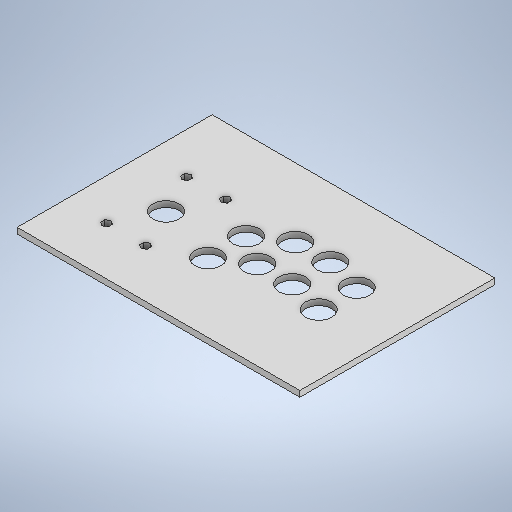
# Autodesk Inventor part: sega_straight_b1_v2
Saved by Autodesk Inventor 2025 (Build 290162010, 162A)
## iProperties
Created: 2022-12-25
Part Number: sega_straight_b1_v2
Material: Generic
Document SubType Name: Modeling
Designer: Bunny
Density: 1 g/cm^3
Appearance: Default
Author: Bunny
Autodesk Inventor part; units mm, degrees
ref_plane "YZ Plane" through (0, 0, 0) normal (1, 0, 0) x (0, 1, 0)
ref_plane "XZ Plane" through (0, 0, 0) normal (0, 1, 0) x (-1, 0, 0)
ref_plane "XY Plane" through (0, 0, 0) normal (0, 0, 1) x (1, 0, 0)
sketch "Sketch1" plane through (0, 0, 0) normal (0, 1, 0) x (-1, 0, 0)
  line L0 (145, -100) -> (-145, -100)
  line L1 (-145, -100) -> (-145, 100)
  line L2 (-145, 100) -> (145, 100)
  line L3 (145, 100) -> (145, -100)
  line L4 (210, 0) -> (-210, 0) projected
  line L5 (0, -140) -> (0, 140) projected
  point P0 (0, 0)
  dimension "d30" = 290
  dimension "d31" = 200
  constraints: 8 end point, 2 parallel, 1 horizontal, 1 perpendicular, 2 other
  measures "d30" distance of L0.start L0.end
  measures "d31" distance of L0.end L1.end
extrude "Extrusion1" add sketch "Sketch1" along normal blind 6
sketch "Sketch2" plane through (0, 6, 0) normal (0, 1, 0) x (1, 0, 0)
  circle A0 centre (-19.75, -29.5) radius 13.5
  circle A1 centre (-82.75, -9.5) radius 13.5
  circle A2 centre (-19.75, 9.5) radius 13.5
  circle A3 centre (46.75, 29.5) radius 13.5
  circle A4 centre (82.75, 20.5) radius 13.5
  circle A5 centre (10.75, 29.5) radius 13.5
  circle A6 centre (10.75, -9.5) radius 13.5
  circle A7 centre (46.75, -9.5) radius 13.5
  circle A8 centre (82.75, -18.5) radius 13.5
  line L0 (-96.25, 43) -> (96.25, 43)
  line L1 (96.25, 43) -> (96.25, -43)
  line L2 (96.25, -43) -> (-96.25, -43)
  line L3 (-96.25, -43) -> (-96.25, 43)
  line L4 (145, 100) -> (-145, 100) projected
  line L5 (145, -100) -> (145, 100) projected
  line L6 (0, 140) -> (0, -140) projected
  line L7 (-210, 0) -> (210, 0) projected
  line L8 (-102.75, 31.5) -> (-62.75, 31.5)
  line L9 (-62.75, 31.5) -> (-62.75, -50.5)
  line L10 (-62.75, -50.5) -> (-102.75, -50.5)
  line L11 (-102.75, -50.5) -> (-102.75, 31.5)
  line L12 (-106.75, 33.8094) -> (-102.75, 36.1188)
  line L13 (-102.75, 36.1188) -> (-98.75, 33.8094)
  line L14 (-98.75, 33.8094) -> (-98.75, 29.1906)
  line L15 (-98.75, 29.1906) -> (-102.75, 26.8812)
  line L16 (-102.75, 26.8812) -> (-106.75, 29.1906)
  line L17 (-106.75, 29.1906) -> (-106.75, 33.8094)
  line L18 (-62.75, 36.1188) -> (-58.75, 33.8094)
  line L19 (-58.75, 33.8094) -> (-58.75, 29.1906)
  line L20 (-58.75, 29.1906) -> (-62.75, 26.8812)
  line L21 (-62.75, 26.8812) -> (-66.75, 29.1906)
  line L22 (-66.75, 29.1906) -> (-66.75, 33.8094)
  line L23 (-66.75, 33.8094) -> (-62.75, 36.1188)
  line L24 (-102.75, -45.8812) -> (-98.75, -48.1906)
  line L25 (-98.75, -48.1906) -> (-98.75, -52.8094)
  line L26 (-98.75, -52.8094) -> (-102.75, -55.1188)
  line L27 (-102.75, -55.1188) -> (-106.75, -52.8094)
  line L28 (-106.75, -52.8094) -> (-106.75, -48.1906)
  line L29 (-106.75, -48.1906) -> (-102.75, -45.8812)
  line L30 (-62.75, -45.8812) -> (-58.75, -48.1906)
  line L31 (-58.75, -48.1906) -> (-58.75, -52.8094)
  line L32 (-58.75, -52.8094) -> (-62.75, -55.1188)
  line L33 (-62.75, -55.1188) -> (-66.75, -52.8094)
  line L34 (-66.75, -52.8094) -> (-66.75, -48.1906)
  line L35 (-66.75, -48.1906) -> (-62.75, -45.8812)
  point P0 (-58.75, 31.5)
  point P1 (-98.75, -50.5)
  point P2 (-106.75, -50.5)
  point P3 (-66.75, -50.5)
  point P4 (-58.75, -50.5)
  dimension "d3" = 27
  dimension "d19" = 30.5
  dimension "d20" = 36
  dimension "d23" = 19
  dimension "d24" = 9
  dimension "d25" = 36
  dimension "d26" = 11
  dimension "d27" = 9
  dimension "d28" = 11
  dimension "d29" = 63
  dimension "d35" = 41
  dimension "d36" = 41
  dimension "d37" = 20
  dimension "d38" = 20
  dimension "d54" = 8
  dimension "d55" = 8
  dimension "d56" = 8
  dimension "d57" = 8
  constraints: 64 end point, 9 centre point, 8 equal radius, 5 midpoint, 5 parallel, 4 coincident, 4 tangent, 4 vertical alignment, 3 horizontal alignment, 2 horizontal, 2 perpendicular, 2 point on line, 54 other
  measures "d3" diameter of A1
  measures "d19" horizontal distance of A0.centre A6.centre
  measures "d20" distance of A7.centre A6.centre
  measures "d23" vertical distance of A6.centre A2.centre
  measures "d24" vertical distance of A8.centre A6.centre
  measures "d25" horizontal distance of A8.centre A7.centre
  measures "d26" vertical distance of A0.centre A8.centre
  measures "d27" vertical distance of A4.centre A5.centre
  measures "d28" vertical distance of A2.centre A4.centre
  measures "d29" horizontal distance of A0.centre A1.centre
  measures "d35" distance from line of L8 A1.centre
  measures "d36" distance from line of L10 A1.centre
  measures "d37" distance from line of L11 A1.centre
  measures "d38" distance from line of L9 A1.centre
  measures "d54" distance between parallel lines of L14 L17
  measures "d55" distance from line of point (-58.75, 31.5) L22
  measures "d56" distance of point (-98.75, -50.5) point (-106.75, -50.5)
  measures "d57" distance of point (-66.75, -50.5) point (-58.75, -50.5)
extrude "Extrusion2" cut sketch "Sketch2" against normal blind 30 contours A0 | A8 | L6 A6 L7 | A6 L6 | L30 L31 L32 L33 L34 L10 L9 | L9 L10 L34 L35 | A1 L7 | L7 A1 | L7 A2 | A2 L7 | L21 L22 L8 L9 | L9 L8 L22 L23 L18 L19 L20 | A4 | A3 | A6 L7 | L7 A7 | A7 L7 | L6 A5 | A5 L6 | L25 L26 L27 L28 L29 L11 L10 | L10 L11 L24 L25 | L14 L15 L11 L8 | L8 L11 L16 L17 L12 L13 L14 picked at (6.7806, -6.3333)
equation "\"d30\" = BoxLength"
equation "\"d31\" = BoxWidth"
equation "\"d3\" = JS_Hole_dia"
equation "\"d36\" = 0.5 * JS_SH_L"
equation "\"d37\" = 0.5 * JS_SH_W"
equation "\"d38\" = 0.5 * JS_SH_W"
equation "\"d55\" = JS_SH_hex_width"
equation "\"d56\" = JS_SH_hex_width"
equation "\"d57\" = JS_SH_hex_width"
equation "\"BoxLength\" = 290"
equation "\"BoxWidth\" = 200"
equation "\"JS_SH_L\" = 82"
equation "\"JS_SH_dia\" = 5"
equation "\"SheetThickness\" = 6"
equation "\"CornerOffset\" = 5"
equation "\"NutS\" = 5.7"
equation "\"NutThreadD2\" = 4.17"
equation "\"SideNutWidth\" = 2.5"
equation "\"JS_Hole_dia\" = 27"
equation "\"JS_SH_hex_width\" = 8"
equation "\"JS_SH_W\" = 40"
body "Solid1"
